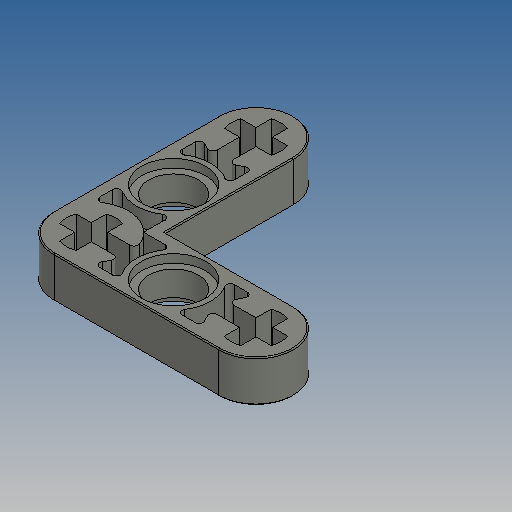
# Autodesk Inventor part: 32056-DkBluishGray
Saved by Autodesk Inventor 2025 (Build 290162010, 162A)
## iProperties
Created: 2012-03-21
Part Number: 32056-DkBluishGray
Document SubType Name: Modeling
Designer: D. Kohfeld
Density: 1.06 g/cm^3
Material: ABS Plastic
Mass: 0.645733 g
Surface Area: 12.2395 cm^2
Volume: 0.609182 cm^3
Appearance: DkBluishGray
Author: D. Kohfeld
Autodesk Inventor part; units mm, degrees
ref_plane "YZ Plane" through (0, 0, 0) normal (1, 0, 0) x (0, 1, 0)
ref_plane "XZ Plane" through (0, 0, 0) normal (0, 1, 0) x (-1, 0, 0)
ref_plane "XY Plane" through (0, 0, 0) normal (0, 0, 1) x (1, 0, 0)
sketch "Sketch1" plane through (0, 0, 0) normal (0, 0, 1) x (1, 0, 0)
  line L0 (3.6, -4.4) -> (3.6, 8)
  line L1 (-3.6, 8) -> (-3.6, -8)
  arc A0 (3.6, 8) -> (-3.6, 8) centre (0, 8) ccw
  circle A1 centre (0, 8) radius 2.4 construction
  circle A2 centre (0, 8) radius 3.2 construction
  circle A3 centre (0, 0) radius 3.2
  circle A4 centre (0, 0) radius 2.4
  line L2 (0, 0) -> (0, 8) construction
  line L3 (-2.5456, 5.4544) -> (-2.5456, 2.5456)
  line L4 (2.5456, 5.4544) -> (2.5456, 2.5456)
  arc A5 (-2.5456, 5.4544) -> (2.5456, 5.4544) centre (0, 8) ccw
  arc A6 (2.5456, 2.5456) -> (-2.5456, 2.5456) centre (0, 0) ccw
  arc A7 (-3.6, -8) -> (0, -11.6) centre (0, -8) ccw
  circle A8 centre (0, -8) radius 3.2 construction
  circle A9 centre (0, -8) radius 2.4 construction
  line L5 (0, 0) -> (0, -8) construction
  line L6 (-2.5456, -2.5456) -> (-2.5456, -5.4544)
  line L7 (2.5456, -2.5456) -> (2.5456, -5.4544)
  arc A10 (-2.5456, -2.5456) -> (2.5456, -2.5456) centre (0, 0) ccw
  arc A11 (2.5456, -5.4544) -> (-2.5456, -5.4544) centre (0, -8) ccw
  line L8 (0.8, 4.49) -> (0.8, 7.2)
  line L9 (0.8, 7.2) -> (2.2627, 7.2)
  line L10 (2.2627, 8.8) -> (0.8, 8.8)
  line L11 (0.8, 8.8) -> (0.8, 10.2627)
  line L12 (-0.8, 10.2627) -> (-0.8, 8.8)
  line L13 (-0.8, 8.8) -> (-2.2627, 8.8)
  line L14 (-2.2627, 7.2) -> (-0.8, 7.2)
  line L15 (-0.8, 7.2) -> (-0.8, 4.49)
  arc A12 (-2.2627, 8.8) -> (-2.2627, 7.2) centre (0, 8) ccw
  arc A13 (0.8, 10.2627) -> (-0.8, 10.2627) centre (0, 8) ccw
  arc A14 (2.2627, 7.2) -> (2.2627, 8.8) centre (0, 8) ccw
  line L16 (-0.8, -10.2627) -> (-0.8, -8.8)
  line L17 (-0.8, -8.8) -> (-2.2627, -8.8)
  line L18 (-2.2627, -7.2) -> (-0.8, -7.2)
  line L19 (-0.8, -7.2) -> (-0.8, -5.7373)
  line L20 (0.8, -5.7373) -> (0.8, -7.2)
  line L21 (0.8, -7.2) -> (3.51, -7.2)
  line L22 (3.51, -8.8) -> (0.8, -8.8)
  line L23 (0.8, -8.8) -> (0.8, -10.2627)
  arc A15 (-2.2627, -7.2) -> (-2.2627, -8.8) centre (0, -8) ccw
  arc A16 (-0.8, -10.2627) -> (0.8, -10.2627) centre (0, -8) ccw
  line L24 (0, -11.6) -> (16, -11.6)
  arc A17 (16, -11.6) -> (16, -4.4) centre (16, -8) ccw
  arc A18 (0.8, -5.7373) -> (-0.8, -5.7373) centre (0, -8) ccw
  line L25 (2.5456, -5.4544) -> (5.4544, -5.4544)
  line L26 (2.5456, -10.5456) -> (5.4544, -10.5456)
  arc A19 (2.5456, -10.5456) -> (2.5456, -5.4544) centre (0, -8) ccw
  circle A20 centre (8, -8) radius 3.2
  circle A21 centre (16, -8) radius 3.2 construction
  circle A22 centre (16, -8) radius 2.4 construction
  line L27 (0, -8) -> (8, -8) construction
  line L28 (8, -8) -> (16, -8) construction
  circle A23 centre (8, -8) radius 2.4
  line L29 (12.49, -7.2) -> (15.2, -7.2)
  line L30 (15.2, -7.2) -> (15.2, -5.7373)
  line L31 (16.8, -5.7373) -> (16.8, -7.2)
  line L32 (16.8, -7.2) -> (18.2627, -7.2)
  line L33 (18.2627, -8.8) -> (16.8, -8.8)
  line L34 (16.8, -8.8) -> (16.8, -10.2627)
  line L35 (15.2, -10.2627) -> (15.2, -8.8)
  line L36 (15.2, -8.8) -> (12.49, -8.8)
  arc A24 (10.5456, -10.5456) -> (10.5456, -5.4544) centre (8, -8) ccw
  arc A25 (13.4544, -5.4544) -> (13.4544, -10.5456) centre (16, -8) ccw
  arc A26 (16.8, -5.7373) -> (15.2, -5.7373) centre (16, -8) ccw
  arc A27 (18.2627, -8.8) -> (18.2627, -7.2) centre (16, -8) ccw
  arc A28 (15.2, -10.2627) -> (16.8, -10.2627) centre (16, -8) ccw
  arc A29 (5.4544, -5.4544) -> (5.4544, -10.5456) centre (8, -8) ccw
  line L37 (10.5456, -5.4544) -> (13.4544, -5.4544)
  line L38 (10.5456, -10.5456) -> (13.4544, -10.5456)
  line L39 (3.6, -4.4) -> (16, -4.4)
  dimension "d8" = 4.8
  dimension "d9" = 6.4
  dimension "d32" = 7.2
  dimension "d34" = 8
  dimension "d52" = 1.6
  dimension "d56" = 1.6
  dimension "d57" = 1.6
  dimension "d58" = 1.6
  constraints: 80 end point, 64 point on circle, 30 centre point, 26 equal radius, 24 equal length, 20 parallel, 16 coincident, 11 perpendicular, 7 tangent, 5 horizontal alignment, 5 vertical alignment, 3 vertical, 2 collinear, 1 concentric
  measures "d8" diameter of A1
  measures "d9" diameter of A2
  measures "d32" diameter of A0
  measures "d34" distance of L2.start L2.end
  measures "d52" distance between parallel lines of L11 L12
  measures "d56" distance between parallel lines of L31 L30
  measures "d57" distance between parallel lines of L20 L19
  measures "d58" distance between parallel lines of L22 L21
extrude "Extrusion1" add sketch "Sketch1" along normal mid plane 4 contours L39 A17 L24 A7 L1 A0 L0 | A3 | A20
extrude "Extrusion9" add sketch "Sketch1" along normal mid plane 0.8 contours A10 L7 A11 L6
sketch "Sketch6" plane through (0, 0, 2) normal (0, 0, 1) x (1, 0, 0)
  circle A0 centre (0, 0) radius 3.1
  circle A1 centre (0, 0) radius 2.4 projected
  circle A2 centre (8, -8) radius 3.1
  circle A3 centre (16, -8) radius 3.1
  arc A4 (16, -11.6) -> (16, -4.4) centre (16, -8) ccw projected
  arc A5 (5.4544, -5.4544) -> (5.4544, -10.5456) centre (8, -8) ccw projected
  dimension "d53" = 6.2
  constraints: 3 centre point, 2 coincident, 2 equal radius, 1 concentric
  measures "d53" diameter of A0
extrude "Extrusion7" cut sketch "Sketch6" against normal blind 0.8 contours A0 | A1 | A2
mirror "Mirror1" about plane through (0, 0, 0) normal (0, 0, 1) of "Extrusion7"
fillet "Fillet1" radius 0.1 14 edges at (0, 11.6, 2) (-3.6, 0, 2) (0, 11.6, -2) (-3.6, 0, -2) (3.6, 1.8, 2) (3.6, 1.8, -2) (19.6, -8, 2) (19.6, -8, -2) (8, -11.6, 2) (-2.5456, -10.5456, 2) (-2.5456, -10.5456, -2) (8, -11.6, -2) (9.8, -4.4, -2) (9.8, -4.4, 2)
fillet "Fillet1" radius 0.4 23 edges at (-2.5456, -2.5456, -1.2) (-2.5456, -2.5456, 1.2) (-2.5456, -5.4544, 1.2) (-2.5456, -5.4544, -1.2) (2.5456, -2.5456, 1.2) (2.5456, -2.5456, -1.2) (-2.5456, 5.4544, 0) (-2.5456, 2.5456, 0) (2.5456, 2.5456, 0) (2.5456, 5.4544, 0) (0.8, 4.49, 0) (-0.8, 4.49, 0) (10.5456, -10.5456, 0) (10.5456, -5.4544, 0) (13.4544, -5.4544, 0) (12.49, -7.2, 0) (12.49, -8.8, 0) (13.4544, -10.5456, 0) (2.5456, -10.5456, 0) (5.4544, -10.5456, 0) (3.51, -8.8, 0) (3.51, -7.2, 0) (5.4544, -5.4544, 0)
equation "\"d8\" = kd"
equation "\"d9\" = tsd"
equation "\"d32\" = tlad"
equation "\"d34\" = lu"
equation "\"d52\" = axlet"
equation "\"d56\" = axlet"
equation "\"d57\" = axlet"
equation "\"d58\" = d57"
equation "\"d14\" = 0.5 * lu"
equation "\"d41\" = tsl"
equation "\"lf\" = 0.1"
equation "\"tf\" = 0.4"
equation "\"kd\" = 4.8"
equation "\"tsd\" = 6.4"
equation "\"tlad\" = 7.2"
equation "\"lu\" = 8"
equation "\"axlet\" = 1.6"
equation "\"tsl\" = 0.8"
body "Solid1"
